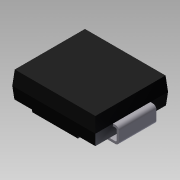
# Autodesk Inventor part: DO-214AB (SMC)
Saved by Autodesk Inventor 2011 (Build 150239000, 239)
## iProperties
Created: 2010-11-23
Part Number: DO-214AB (SMC)
Document SubType Name: Modeling
Designer: abbath
Density: 1 g/cm^3
Mass: 0.103526 g
Surface Area: 1.84787 cm^2
Volume: 0.103526 cm^3
Author: abbath
Autodesk Inventor part; units mm, degrees
sketch "Эскиз1" plane through (0, 0, 0) normal (0, 0, 1) x (1, 0, 0)
  line L0 (-3.555, 3.11) -> (3.555, 3.11)
  line L1 (3.555, 3.11) -> (3.555, -3.11)
  line L2 (3.555, -3.11) -> (-3.555, -3.11)
  line L3 (-3.555, -3.11) -> (-3.555, 3.11)
  point P0 (0, 0)
  dimension "d0" = 3.555
  dimension "d1" = 3.11
  dimension "d2" = 7.11
  dimension "d3" = 6.22
  constraints: 8 end point, 2 parallel, 1 horizontal, 1 perpendicular
  measures "d0" distance from line of L3 point (0, 0)
  measures "d1" distance from line of L0 point (0, 0)
  measures "d2" distance between parallel lines of L1 L3
  measures "d3" distance between parallel lines of L2 L0
extrude "Выдавливание1" add sketch "Эскиз1" along normal blind 2.62
sketch "Эскиз4" plane through (-3.555, -3.11, 0) normal (0, -1, 0) x (1, 0, 0)
  line L0 (7.11, 2.62) -> (0, 2.62) projected
  line L1 (0, 0) -> (0, 2.62) projected
  line L2 (7.11, 0) -> (0, 0) projected
  line L3 (7.11, 0) -> (7.11, 2.62) projected
  line L4 (0.1057, 2.62) -> (0, 1.4115)
  line L5 (0, 1.4115) -> (0.088, 0.406)
  line L6 (7.0043, 2.62) -> (7.11, 1.4115)
  line L7 (7.11, 1.4115) -> (7.022, 0.406)
  line L8 (0.088, 0.406) -> (1.6, 0.406)
  line L9 (1.6, 0.406) -> (1.6, 0.203)
  line L10 (1.6, 0.203) -> (5.51, 0.203)
  line L11 (5.51, 0.203) -> (5.51, 0.406)
  line L12 (5.51, 0.406) -> (7.022, 0.406)
  point P0 (3.555, 0)
  dimension "d24" = 0.203
  dimension "d25" = 0.203
  dimension "d26" = 1.6
  dimension "d27" = 1.6
  dimension "d28" = 1.2085
  dimension "d29" = 1.2085
  dimension "d30" = 1.2085
  dimension "d31" = 1.2085
  dimension "d32" = 5
  dimension "d33" = 5
  dimension "d34" = 5
  dimension "d35" = 5
  constraints: 18 end point, 4 point on line, 3 perpendicular, 2 parallel, 1 collinear
  measures "d24" distance between parallel lines of L2 L10
  measures "d25" distance between parallel lines of L8 L10
  measures "d26" distance between parallel lines of L1 L9
  measures "d27" distance between parallel lines of L3 L11
  measures "d28" distance from line of L4.end L0
  measures "d29" distance from line of L4.end L10
  measures "d30" distance from line of L6.end L0
  measures "d31" distance from line of L6.end L10
  measures "d32" angle of L1 L4
  measures "d33" angle of L3 L6
  measures "d34" angle of L3 L7
  measures "d35" angle of L1 L5
extrude "Выдавливание3" cut sketch "Эскиз4" against normal through all contours L3 L6 L0 | L3 L2 L1 L5 L8 L9 L10 L11 L12 L7 | L4 L1 L0
ref_plane "РабПлоскость1" through (3.555, 0, 1.4115) normal (1, 0, 0) x (0, 1, 0)
sketch "Эскиз5" plane through (3.555, 0, 1.4115) normal (1, 0, 0) x (0, 1, 0)
  line L0 (3.11, 1.2085) -> (3.11, 0) projected
  line L1 (-3.11, 1.2085) -> (3.11, 1.2085) projected
  line L2 (-3.11, 0) -> (-3.11, 1.2085) projected
  line L3 (-3.11, 0) -> (3.11, 0) projected
  line L4 (3.11, 0) -> (3.11, -1.0055) projected
  line L5 (-3.11, 0) -> (3.11, 0) projected
  line L6 (-3.11, -1.0055) -> (-3.11, 0) projected
  line L7 (-3.11, -1.0055) -> (3.11, -1.0055) projected
  line L8 (-3.11, 0) -> (-3.0043, 1.2085)
  line L9 (3.11, 0) -> (3.0043, 1.2085)
  line L10 (-3.0043, 1.2085) -> (-3.11, 1.2085)
  line L11 (-3.11, 1.2085) -> (-3.11, 0)
  line L12 (3.11, 0) -> (3.11, 1.2085)
  line L13 (3.11, 1.2085) -> (3.0043, 1.2085)
  line L14 (3.11, -1.0055) -> (3.11, -1.2085) projected
  line L15 (-3.11, -1.0055) -> (3.11, -1.0055) projected
  line L16 (-3.11, -1.2085) -> (-3.11, -1.0055) projected
  line L17 (-3.11, -1.2085) -> (3.11, -1.2085) projected
  line L18 (-3.11, 0) -> (-3.0043, -1.2085)
  line L19 (-3.0043, -1.2085) -> (-3.11, -1.2085)
  line L20 (-3.11, -1.2085) -> (-3.11, 0)
  line L21 (3.11, 0) -> (3.0043, -1.2085)
  line L22 (3.0043, -1.2085) -> (3.11, -1.2085)
  line L23 (3.11, -1.2085) -> (3.11, 0)
  point P0 (0, -1.4115)
  dimension "d39" = 5
  dimension "d40" = 5
  dimension "d43" = 5
  dimension "d44" = 5
  constraints: 24 end point, 5 perpendicular, 4 point on line, 3 collinear
  measures "d39" angle of L8 L2
  measures "d40" angle of L0 L9
  measures "d43" angle of L21 L23
  measures "d44" angle of L18 L20
extrude "Выдавливание4" cut sketch "Эскиз5" against normal through all contours L0 L9 L1 | L4 L7 L21 | L18 L7 L6 | L2 L1 L8 | L14 L17 L21 L7 | L7 L18 L17 L16
ref_plane "РабПлоскость10" through (3.555, 0, 1.4115) normal (0, 1, 0) x (-1, 0, 0)
ref_plane "РабПлоскость8" through (3.555, -3.11, 1.4115) normal (0, 1, 0) x (-1, 0, 0)
ref_plane "РабПлоскость9" through (0, 3.11, 1.4115) normal (0, 1, 0) x (-1, 0, 0)
sketch "Эскиз7" plane through (3.555, 0, 1.4115) normal (0, 1, 0) x (-1, 0, 0)
  line L0 (0.1057, 1.2085) -> (0, 0) projected
  line L1 (7.0043, 1.2085) -> (0.1057, 1.2085) projected
  line L2 (7.11, 0) -> (7.0043, 1.2085) projected
  line L3 (0, 0) -> (7.11, 0) projected
  line L4 (0, 0) -> (0.088, -1.0055) projected
  line L5 (0, 0) -> (7.11, 0) projected
  line L6 (7.022, -1.0055) -> (7.11, 0) projected
  line L7 (5.51, -1.0055) -> (7.022, -1.0055) projected
  line L8 (5.51, -1.2085) -> (5.51, -1.0055) projected
  line L9 (1.6, -1.2085) -> (5.51, -1.2085) projected
  line L10 (1.6, -1.0055) -> (1.6, -1.2085) projected
  line L11 (0.088, -1.0055) -> (1.6, -1.0055) projected
  line L12 (3.555, -1.4115) -> (3.555, 2.1644) construction
  line L13 (-0.51, -0.3) -> (-0.51, -1.1115)
  line L14 (1.01, -1.4115) -> (-0.21, -1.4115)
  line L15 (1.01, -1.2115) -> (1.01, -1.4115)
  line L16 (1.01, -1.2115) -> (-0.21, -1.2115)
  line L17 (0, 0) -> (-0.21, 0)
  line L18 (0, 0) -> (0.0175, -0.2)
  line L19 (0.0175, -0.2) -> (-0.21, -0.2)
  line L20 (-0.31, -0.3) -> (-0.31, -1.1115)
  arc A0 (-0.31, -1.1115) -> (-0.21, -1.2115) centre (-0.21, -1.1115) ccw
  arc A1 (-0.21, -0.2) -> (-0.31, -0.3) centre (-0.21, -0.3) ccw
  arc A2 (-0.51, -1.1115) -> (-0.21, -1.4115) centre (-0.21, -1.1115) ccw
  arc A3 (-0.21, 0) -> (-0.51, -0.3) centre (-0.21, -0.3) ccw
  line L21 (3.555, -1.4115) -> (1.6, -1.4115) construction
  dimension "d62" = 4.065
  dimension "d64" = 1.52
  dimension "d65" = 0.2
  dimension "d66" = 0.2
  dimension "d67" = 0.2
  dimension "d68" = 0.2
  dimension "d69" = 0.2
  constraints: 21 end point, 8 point on circle, 6 perpendicular, 6 tangent, 4 centre point, 3 parallel, 2 coincident, 1 collinear, 1 point on line
  measures "d62" distance between parallel lines of L13 L12
  measures "d64" distance between parallel lines of L15 L13
  measures "d65" distance between parallel lines of L14 L16
  measures "d66" distance between parallel lines of L19 L17
  measures "d67" distance between parallel lines of L13 L20
  measures "d68" diameter of A0
  measures "d69" diameter of A1
extrude "Выдавливание6" add sketch "Эскиз7" along normal mid plane 3.2 contours L4 L19 A1 L20 A0 L16 L15 L14 A2 L13 A3 L17
ref_plane "РабПлоскость13" through (0, -3.11, 1.4115) normal (-1, 0, 0) x (0, -1, 0)
ref_plane "РабПлоскость11" through (3.555, 0, 1.4115) normal (1, 0, 0) x (0, 1, 0)
ref_plane "РабПлоскость12" through (-3.555, -3.11, 1.4115) normal (-1, 0, 0) x (0, -1, 0)
mirror "Зеркальное отражение2" about plane through (0, -3.11, 1.4115) normal (-1, 0, 0) of "Выдавливание6"
equation "\"d0\" = 0.5 * d2"
equation "\"d1\" = 0.5 * d3"
equation "\"d25\" = d24"
equation "\"d27\" = d26"
equation "\"d28\" = d29"
equation "\"d30\" = d31"
